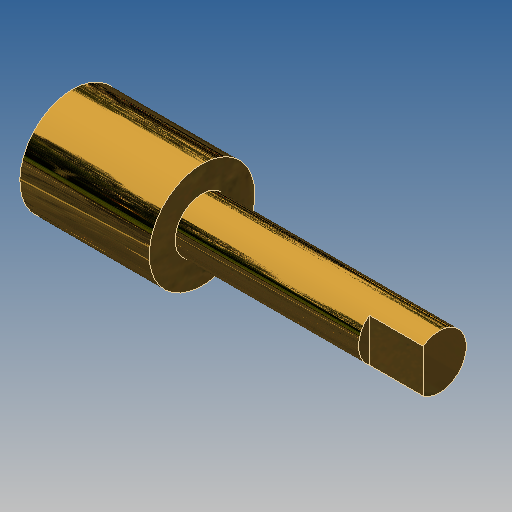
# Autodesk Inventor part: M000
Saved by Autodesk Inventor 2017 (Build 210142000, 142)
## iProperties
Created: 2018-10-12
Part Number: M000
Material: Laiton / Messing
Document SubType Name: Modeling
Designer: Gilles Mottiez
Density: 8.47 g/cm^3
Appearance: Laiton - Satiné
Description: Arbre de transmission
Mass: 10.2066 g
Surface Area: 9.62593 cm^2
Volume: 1.20502 cm^3
Author: Gilles Mottiez
Autodesk Inventor part; units mm, degrees
ref_plane "YZ Plane" through (0, 0, 0) normal (1, 0, 0) x (0, 1, 0)
ref_plane "XZ Plane" through (0, 0, 0) normal (0, 1, 0) x (-1, 0, 0)
ref_plane "XY Plane" through (0, 0, 0) normal (0, 0, 1) x (1, 0, 0)
sketch "Sketch1" plane through (0, 0, 0) normal (0, 0, 1) x (1, 0, 0)
  line L0 (0, 0) -> (34, 0) construction
  line L1 (0, 0) -> (0, 4.9) construction
  line L2 (0, 4.9) -> (12, 4.9)
  line L3 (12, 4.9) -> (12, 2.5)
  line L4 (12, 2.5) -> (34, 2.5)
  line L5 (34, 2.5) -> (34, 0) construction
  line L6 (0, 4.9) -> (0, 2.45)
  line L7 (0, 2.45) -> (6, 2.45)
  line L8 (6, 2.45) -> (6, 0)
  line L9 (34, 2.5) -> (34, 0)
  line L10 (6, 0) -> (34, 0)
  dimension "d0" = 34
  dimension "d3" = 12
  dimension "d4" = 9.8
  dimension "d5" = 4.9
  dimension "d6" = 6
  dimension "d7" = 5
  constraints: 22 end point, 5 perpendicular, 3 horizontal, 1 collinear, 1 midpoint, 1 point on line, 1 vertical
  measures "d0" distance of L0.start L0.end
  measures "d3" distance of L1.end L2.end
  measures "d4" diameter of L2 L10
  measures "d5" diameter of L7 L10
  measures "d6" distance between parallel lines of L1 L8
  measures "d7" diameter of L4 L10
revolve "Révolution1" add sketch "Sketch1" angle 360 about axis through (6, 0, 0) along (1, 0, 0)
sketch "Esquisse2" plane through (34, 0, 0) normal (1, 0, 0) x (0, 0, -1)
  circle A0 centre (0, 0) radius 2.5 construction
  line L0 (-1.5, -2) -> (-1.5, 2)
  arc A1 (-1.5, 2) -> (-1.5, -2) centre (0, 0) ccw
  dimension "d9" = 1.5
  constraints: 4 point on circle, 2 end point, 1 centre point, 1 concentric, 1 vertical
  measures "d9" distance from line of point (0, 0) L0
extrude "Extrusion1" cut sketch "Esquisse2" against normal blind 5
ref_plane "Plan de construction2" through (6, 0, -4.9) normal (0, 0, -1) x (-1, 0, 0)
ref_plane "Plan de construction1" through (6, 0, 4.9) normal (0, 0, 1) x (1, 0, 0)
sketch "Esquisse4" plane through (6, 0, -4.9) normal (0, 0, -1) x (-1, 0, 0)
  line L0 (6, 4.9) -> (6, -4.9) construction
  point P0 (6, 0)
  point P1 (4, 0)
  dimension "d20" = 2
  constraints: 1 horizontal alignment
  measures "d20" distance from line of L0 point (4, 0)
hole "Perçage2" at (2, 0, -4.9) direction (0, 0, 1) diameter 1.567 depth 5 tip angle 118 countersink diameter 2.2 countersink angle 90 thread size "M2x0.4" class "6H" standard "ISO Metric profile"
